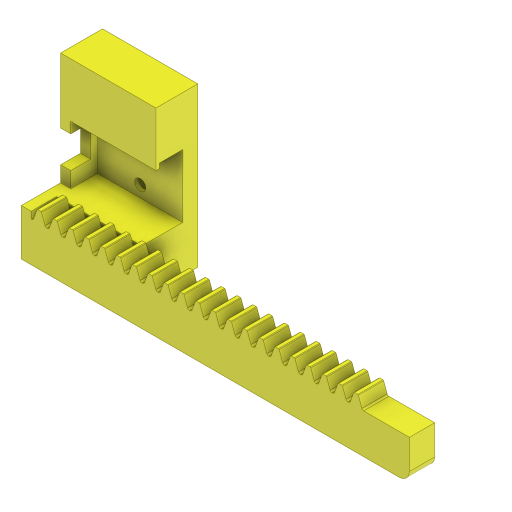
# Autodesk Inventor part: linear-gear
Saved by Autodesk Inventor 2023 (Build 270158000, 158)
## iProperties
Category: PARTsolutions
Company: MISUMI
Created: 2024-11-28
Part Number: linear-gear
Material: ABS プラスチック
Catalog Web Link: www.cadenas.de
Description: RGEAL, RGEABL, RGEASL, RGEAML-Rack Gears L Dimension Configurable (One End Machined) - Pressure Angle 20 - Hole Position Configurable
Vendor: MISUMI
Document SubType Name: Modeling
Designer: psAdmin
Manufacturer: MISUMI
Mass: 2.6861 g
Surface Area: 16.0116 cm^2
Volume: 2.6861 cm^3
Density: 1.06 g/cm^3
Appearance: 黄
PSOL_IDENT_0: {$CADENAS_DATA/23d-libs/misumi/metric/54_spur_gears/rgeasl.prj},239 {VTYP=3D},{NB=RGEASL1.0N-30},{LI
PSOL_IDENT_1: NA=RGEASL1.0N-30},{NN=RGEAL, RGEABL, RGEASL, RGEAML},{DATE=29.05.2023 09:31:20},{GEOMDATE=18.01.2021
PSOL_IDENT_2: 08:14:07},{VERSION=},{LINEID=30},{WBVAR=MAT,HM,L,A,B,C,D,ALT1,ALT2,MS,ALT3,TPC},{WBNUMERIC=L,A,B,C,
PSOL_IDENT_3: D,MS}  {NB=RGEASL1.0N-30},{LINA=RGEASL1.0N-30},{KT=DUMMY},{PN=RGEASL1.0N-30},{MAT=3},{MATALG='1','Fr
PSOL_IDENT_4: ee-Cutting Brass Bar','2','1045 Carbon Steel Equivalent','3','304 Stainless Steel','4','MC Nylon', '
PSOL_IDENT_5: 5','Polyacetal' },{TYPE=RGEASL},{MOD=1.0},{MOD1=1.0},{HM=N},{HMALG='N','No Hole Machining','HT','Bac
PSOL_IDENT_6: k Tapped','ST','Side Tapped','Z','Side Counterbore'},{L=30},{LALG=[20:980/1]},{DD21=6.5},{M12=3},{M1=
PSOL_IDENT_7: 0},{A=0},{AALG=0},{AMIN=0},{AMAX=25},{B=0},{BALG=0},{BMIN=0},{BMAX=25},{C=0},{CALG=0},{CMIN=0},{CMAX=
PSOL_IDENT_8: 25},{D=0},{DALG=0},{DMIN=0},{DMAX=25},{PITCH=3.142},{W=10},{H=10},{HH=9.0},{DD1=3.5},{DD2=6.5},{Z1=3
PSOL_IDENT_9: .5},{M=-},{ALT1= },{ALT1ALG= ' ', 'w/o MC (One End Female Thread Machining)', 'MC', 'with MC (One En
PSOL_IDENT_10: d Female Thread Machining)' },{ALT2= },{ALT2ALG= ' ', 'w/o WMC (Both Ends Female Thread Machining)',
PSOL_IDENT_11: 'WMC', 'with WMC (Both Ends Female Thread Machining)' },{ALT2ALGMAX=30},{MS=0},{MSALG=0},{ALT3=},{A
PSOL_IDENT_12: LT3ALG= '','Not applicable' },{TPC=N/A},{TPCA= 'N/A' },{APN=},{BPN=},{CPN=},{DPN=},{MCPN=},{WMCPN=},
PSOL_IDENT_13: {MSPN=},{ALT3PN=},{TED=2.250},{SP=1.571},{PFP=0.38},{HAP=1},{HFP=1.25},{DEG1=20},{NN=9},{L3=1.14947}
PSOL_IDENT_14: ,{NN1=10},{MC3DL1=0.000},{MC3DL2=0.000},{MCCIF3D=2.000}
NB: RGEASL1.0N-30
NN: RGEAL, RGEABL, RGEASL, RGEAML
NT: Rack Gears L Dimension Configurable (One End Machined) - Pressure Angle 20 - Hole Position Configurable
NBSYN: $PN.
LINA: RGEASL1.0N-30
CATALOG: Misumi
PN: RGEASL1.0N-30
MAT: 304 Stainless Steel
MOD: 1.0
HM: No Hole Machining
L: 30
A: 0
B: 0
C: 0
D: 0
PITCH: 3.142
W: 10
H: 10
HH: 9
DD1: 3.5
DD2: 6.5
Z1: 3.5
M: -
ALT1: w/o MC (One End Female Thread Machining)
ALT2: w/o WMC (Both Ends Female Thread Machining)
MS: 0
ALT3: Not applicable
TPC: N/A
SUPPLIER: MISUMI
ARTICLENO: RGEASL1.0N-30
BOMINFO: RGEASL1.0N-30
CREATOR: CADENAS GmbH
Title: RGEASL1.0N-30
Author: Cadenas PARTsolutions
Comments: Rack Gears L Dimension Configurable (One End Machined) - Pressure Angle 20 - Hole Position Configurable
Autodesk Inventor part; units mm, degrees
ref_plane "YZ Plane" through (0, 0, 0) normal (1, 0, 0) x (0, 1, 0)
ref_plane "XZ Plane" through (0, 0, 0) normal (0, 1, 0) x (-1, 0, 0)
ref_plane "XY Plane" through (0, 0, 0) normal (0, 0, 1) x (1, 0, 0)
sketch "Sketch_1" plane through (0, 0, 0) normal (0, 0, 1) x (1, 0, 0)
  line L0 (0, 10) -> (0, -0.125)
  line L1 (0, -0.125) -> (75, -0.125)
  line L2 (75, -0.125) -> (75, 10)
  line L3 (75, 10) -> (0, 10)
  dimension "d13" = 10.125
  dimension "d14" = 75
  constraints: 8 end point, 2 horizontal, 2 vertical
  measures "d13" distance of L0.start L0.end
  measures "d14" distance of L2.end L0.start
extrude "Extrusion1" add sketch "Sketch_1" along normal blind 5
sketch "_____14" plane through (0, 0, 0) normal (0, 0, 1) x (1, 0, 0)
  line L0 (-1.1495, 10) -> (-0.4215, 8)
  arc A0 (-0.4215, 8) -> (-0.0645, 7.75) centre (-0.0645, 8.13) ccw
  line L1 (-0.0645, 7.75) -> (0.0645, 7.75)
  arc A1 (0.0645, 7.75) -> (0.4215, 8) centre (0.0645, 8.13) ccw
  line L2 (0.4215, 8) -> (1.1495, 10)
  line L3 (1.1495, 10) -> (-1.1495, 10)
  constraints: 8 end point, 4 point on circle, 2 centre point
extrude "Extrusion2" cut sketch "_____14" along normal blind 10
pattern_linear "Rectangular Pattern1" count 22 spacing 3.142 along (1, 0, 0) of "Extrusion2"
chamfer "面取り1" distance 0.1 angle 45 42 edges at (1.1495, 10, 2.5) (1.9925, 10, 2.5) (4.2915, 10, 2.5) (5.1345, 10, 2.5) (7.4335, 10, 2.5) (8.2765, 10, 2.5) (10.5755, 10, 2.5) (11.4185, 10, 2.5) (13.7175, 10, 2.5) (14.5605, 10, 2.5) (16.8595, 10, 2.5) (17.7025, 10, 2.5) (20.0015, 10, 2.5) (20.8445, 10, 2.5) (23.1435, 10, 2.5) (23.9865, 10, 2.5) (26.2855, 10, 2.5) (27.1285, 10, 2.5) (29.4275, 10, 2.5) (30.2705, 10, 2.5) (32.5695, 10, 2.5) (33.4125, 10, 2.5) (35.7115, 10, 2.5) (36.5545, 10, 2.5) (38.8535, 10, 2.5) (39.6965, 10, 2.5) (41.9955, 10, 2.5) (42.8385, 10, 2.5) (45.1375, 10, 2.5) (45.9805, 10, 2.5) (48.2795, 10, 2.5) (49.1225, 10, 2.5) (51.4215, 10, 2.5) (52.2645, 10, 2.5) (54.5635, 10, 2.5) (55.4065, 10, 2.5) (57.7055, 10, 2.5) (58.5485, 10, 2.5) (60.8475, 10, 2.5) (61.6905, 10, 2.5) (63.9895, 10, 2.5) (64.8325, 10, 2.5)
sketch "スケッチ5" plane through (0, -0.125, 0) normal (-1, 0, 0) x (0, 0, 1)
  line L0 (0, 0) -> (-11.1, 0)
  line L1 (-11.1, 0) -> (-11.1, 31.5)
  line L2 (-11.1, 31.5) -> (-2.8, 31.5)
  line L3 (-2.8, 31.5) -> (-2.8, 20.75)
  line L4 (-2.8, 20.75) -> (-3.5, 20.75)
  line L5 (-3.5, 20.75) -> (-3.5, 21.7)
  line L6 (-3.5, 21.7) -> (-8.1, 21.7)
  line L7 (-8.1, 21.7) -> (-8.1, 9.2)
  line L8 (-8.1, 9.2) -> (0, 9.2)
  line L9 (0, 7.875) -> (0, 0) projected
  line L10 (0, 0) -> (5, 0) projected
  line L11 (5, 7.875) -> (5, 0) projected
  line L12 (0, 7.875) -> (5, 7.875) projected
  line L13 (0, 9.2) -> (0, 7.875)
  point P0 (-5.55, 0)
  point P1 (-3.5, 21.225)
  dimension "d37" = 12.5
  dimension "d43" = 3
  dimension "d44" = 10.75
  dimension "d100" = 7.6
  dimension "d118" = 31.5
  dimension "d121" = 9.2
  dimension "d130" = 0.7
  dimension "d131" = 2.8
  constraints: 20 end point, 9 perpendicular, 2 midpoint, 1 collinear, 1 horizontal, 1 point on line
  measures "d37" distance of L6.end L7.end
  measures "d43" distance between parallel lines of L7 L1
  measures "d44" distance of L2.end L3.end
  measures "d100" distance between parallel lines of L5 L1
  measures "d118" distance between parallel lines of L0 L2
  measures "d121" distance from line of point (-5.55, 0) L8
  measures "d130" distance from line of point (-3.5, 21.225) L3
  measures "d131" distance between parallel lines of L9 L3
extrude "押し出し7" add sketch "スケッチ5" against normal blind 16.9 contours L0 L1 L2 L3 L4 L5 L6 L7 L8 L13 L9
sketch "スケッチ9" plane through (0, -0.125, 5) normal (-1, 0, 0) x (0, 0, 1)
  line L0 (-16.1, 31.5) -> (-16.1, 0) projected
  line L1 (-16.1, 31.5) -> (-16.1, 0)
  line L2 (-16.1, 0) -> (0, 0) projected
  line L3 (-16.1, 0) -> (-5, 0)
  line L4 (-5, 0) -> (-5, 9.2) projected
  line L5 (-7.8, 12.3) -> (-11.75, 12.3)
  line L6 (-11.75, 12.3) -> (-11.75, 18.6)
  line L7 (-11.75, 18.6) -> (-7.8, 18.6)
  line L8 (-7.8, 18.6) -> (-7.8, 31.5)
  line L9 (-16.1, 31.5) -> (-7.8, 31.5) projected
  line L10 (-7.8, 20.75) -> (-7.8, 31.5) projected
  line L11 (-13.1, 9.2) -> (-13.1, 21.7) projected
  line L12 (0, 7.875) -> (0, 0) projected
  line L13 (-5, 8.125) -> (-5, 10.031) projected
  line L14 (-5, 8.125) -> (-5, 9.2) projected
  line L15 (-5, 9.2) -> (0, 9.2)
  line L16 (-5, 7.875) -> (0, 7.875) projected
  line L17 (0, 9.2) -> (0, 7.875)
  line L18 (-7.8, 12.3) -> (-7.8, 9.2)
  line L19 (-13.1, 9.2) -> (-5, 9.2) projected
  point P0 (-11.75, 15.45)
  dimension "d124" = 1.35
  dimension "d125" = 6.3
  dimension "d126" = 16.05
  constraints: 19 end point, 3 perpendicular, 2 collinear, 2 point on line, 2 vertical, 1 horizontal, 1 midpoint
  measures "d124" distance between parallel lines of L11 L6
  measures "d125" distance of L5.end L6.end
  measures "d126" distance from line of L9 point (-11.75, 15.45)
extrude "押し出し10" add sketch "スケッチ9" along normal blind 2
sketch "スケッチ10" plane through (16.9, -0.125, -11.1) normal (0, 0, -1) x (-1, 0, 0)
  line L0 (16.9, 9.2) -> (16.9, 21.7) projected
  line L1 (0, 31.5) -> (18.9, 31.5) projected
  line L2 (0, 0) -> (18.9, 0) projected
  line L3 (16.9, 9.2) -> (0, 9.2) projected
  point P0 (16.9, 0.125)
  point P1 (8.4, 19.45)
  point P2 (8.4, 11.45)
  dimension "d88" = 8
  dimension "d90" = 8.5
  dimension "d91" = 8.5
  dimension "d133" = 2.25
  measures "d88" distance of point (8.4, 11.45) point (8.4, 19.45)
  measures "d90" distance from line of point (8.4, 11.45) L0
  measures "d91" distance from line of L0 point (8.4, 19.45)
  measures "d133" distance from line of point (8.4, 11.45) L3
hole "穴1" at (8.5, 19.325, -11.1) at (8.5, 11.325, -11.1) direction (0, 0, 1) diameter 2.2 depth 8 tip angle 118 counterbore diameter 4.2 counterbore depth 2.2
sketch "スケッチ11" plane through (16.9, -0.125, -11.1) normal (0, 0, -1) x (-1, 0, 0)
  circle A0 centre (8.9, 4) radius 2.25
  line L0 (0, 0) -> (18.9, 0) projected
  line L1 (18.9, 31.5) -> (18.9, 0) projected
  circle A1 centre (8.9, 27.5) radius 2.25
  line L2 (0, 0) -> (0, 31.5) projected
  point P0 (16.9, 0.125)
  dimension "d107" = 10
  dimension "d102" = 4.5
  dimension "d103" = 4
  dimension "d110" = 23.5
  dimension "d129" = 8.9
  constraints: 2 centre point, 1 horizontal, 1 vertical, 2 other
  measures "d102" diameter of A0
  measures "d103" distance from line of L0 A0.centre
  measures "d110" distance of A0.centre A1.centre
  measures "d129" distance from line of L2 A1.centre
extrude "押し出し11" cut sketch "スケッチ11" against normal blind 6
sketch "スケッチ12" plane through (0, 0, 0) normal (0, 0, -1) x (-1, 0, 0)
  line L0 (-66.0465, 7.75) -> (-65.9175, 7.75) projected
  line L1 (-65.982, 7.75) -> (-75, 7.75)
  line L2 (-75, -0.125) -> (-75, 10) projected
  line L3 (-75, 10) -> (-67.1315, 10) projected
  line L4 (-66.4035, 8) -> (-67.1315, 10) projected
  arc A0 (-66.4035, 8) -> (-66.0465, 7.75) centre (-66.0465, 8.13) ccw projected
  point P0 (0, 0)
  point P1 (-67.2315, 10)
  point P2 (-67.0973, 9.906)
  constraints: 2 end point, 1 horizontal, 1 midpoint, 1 point on line
extrude "押し出し12" cut sketch "スケッチ12" against normal blind 5
fillet "フィレット1" radius 2 1 edges at (75, -0.125, 2.5)
body "Solid1"
